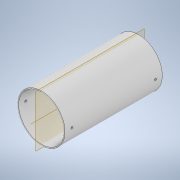
# Autodesk Inventor part: EimarTube
Saved by Autodesk Inventor 2021.2 (Build 252289000, 289)
## iProperties
Created: 2022-10-01
Part Number: EimarTube
Material: Типовые
Document SubType Name: Modeling
Designer: Andrei
Density: 1 g/cm^3
Appearance: По умолчанию
Author: Andrei
Autodesk Inventor part; units mm, degrees
ref_plane "XZ Plane" through (0, 0, 0) normal (0, 1, 0) x (-1, 0, 0)
ref_plane "XY Plane" through (0, 0, 0) normal (0, 0, 1) x (1, 0, 0)
sketch "Эскиз1" plane through (0, 0, 0) normal (0, 0, 1) x (1, 0, 0)
  circle A0 centre (0, 0) radius 46.1
  circle A1 centre (0, 0) radius 48.1
  dimension "d0" = 92.2
  dimension "d1" = 96.2
  constraints: 2 centre point, 2 coincident
  measures "d0" diameter of A0
  measures "d1" diameter of A1
extrude "Выдавливание1" add sketch "Эскиз1" along normal blind 200
fillet "Сопряжение1" radius 1 4 edges at (-48.1, 0, 200) (-46.1, 0, 200) (-48.1, 0, 0) (-46.1, 0, 0)
sketch "Эскиз2" plane through (0, 0, 0) normal (1, 0, 0) x (0, 1, 0)
  circle A0 centre (0, 15) radius 2
  circle A1 centre (0, 185) radius 2
  point P0 (0, 0)
  dimension "d5" = 4
  dimension "d6" = 4
  dimension "d7" = 15
  dimension "d8" = 185
  constraints: 2 centre point
  measures "d5" diameter of A1
  measures "d6" diameter of A0
  measures "d7" distance of A0.centre point (0, 0)
  measures "d8" distance of point (0, 0) A1.centre
hole "Отверстие1" at (0, 0, 185) at (0, 0, 15) direction (-1, 0, 0) diameter 4 end through all both
equation "\"d0\" = dInternal"
equation "\"d1\" = dInternal + wallThickness"
equation "\"d2\" = tubeHeight"
equation "\"d4\" = 0.25 * wallThickness"
equation "\"d5\" = dHole"
equation "\"d6\" = dHole"
equation "\"d7\" = distanceHoles"
equation "\"d8\" = tubeHeight - distanceHoles"
equation "\"d9\" = dHole"
equation "\"dInternal\" = 92.2"
equation "\"wallThickness\" = 4"
equation "\"tubeHeight\" = 200"
equation "\"dHole\" = 4"
equation "\"distanceHoles\" = 15"
